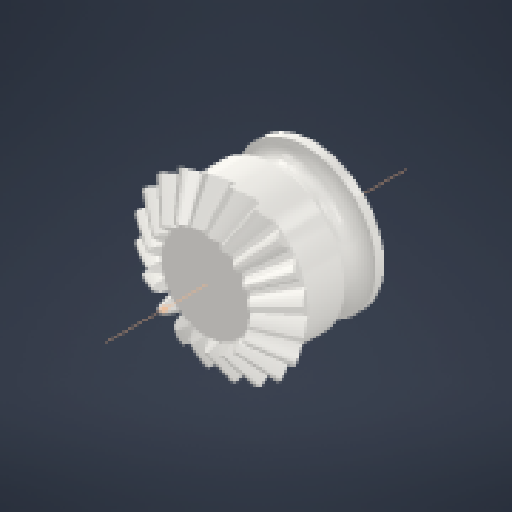
# Autodesk Inventor part: Bevel Gear2
Saved by Autodesk Inventor 2023.4 (Build 274418000, 418)
## iProperties
CustomPartVersion: 1
Created: 2025-10-03
Part Number: Bevel Gear2
Material: Steel, Mild
Document SubType Name: Modeling
Designer: Malthe Sennels
Categories: <?xml version="1.0" encoding="UTF-16"?> <MemberInstance><Categories><FamilyTemplate><FamilyTemplateParameter ValueType="xs:double" Id="1" ObjectReferenceKey="da_z" ObjectType="kUserParameterObject"/><FamilyTemplateParameter ValueType="xs:double" Id="2" ObjectReferenceKey="da_b" ObjectType="kUserParameterObject"/><FamilyTemplateParameter ValueType="xs:double" Id="3" ObjectReferenceKey="da_beta" ObjectType="kUserParameterObject"/><FamilyTemplateParameter ValueType="xs:double" Id="4" ObjectReferenceKey="da_dae" ObjectType="kUserParameterObject"/><FamilyTemplateParameter ValueType="xs:double" Id="5" ObjectReferenceKey="da_ve" ObjectType="kUserParameterObject"/><FamilyTemplateParameter ValueType="xs:double" Id="6" ObjectReferenceKey="da_omega" ObjectType="kUserParameterObject"/><FamilyTemplateParameter ValueType="xs:string" Id="7" ObjectReferenceKey="EAIAABAAAAAAHwAAAAAAAIAAAAAAAAAA" ObjectType="83914240" SubObjectId="SurfaceGeometry"/></FamilyTemplate><ParamToTemplateMap><ParamToTemplate CategoryParameter="//CategoryParameter[@InternalName='046C89C9-8512-4d59-83FE-43B91F4F132A']" TemplateParameter="1"/><ParamToTemplate CategoryParameter="//CategoryParameter[@InternalName='2552DF32-E462-4b46-AEBF-C6C7768E72AC']" TemplateParameter="2"/><ParamToTemplate CategoryParameter="//CategoryParameter[@InternalName='C9EE641D-15FC-4fae-A226-E94C4372FDD7']" TemplateParameter="3"/><ParamToTemplate><ParamToTemplate CategoryParameter="//CategoryParameter[@InternalName='00B6519A-459B-49c7-AD84-2E56D39A5744']" ConstantValue="-0.000000"/></ParamToTemplate><ParamToTemplate><ParamToTemplate CategoryParameter="//CategoryParameter[@InternalName='04B31F0E-C7A6-4894-AA32-9629BEFACF47']" ConstantValue="1.000000"/></ParamToTemplate><ParamToTemplate><ParamToTemplate CategoryParameter="//CategoryParameter[@InternalName='43CBEC2E-7847-49e7-A936-2F7889FCB2D9']" ConstantValue="0.200000"/></ParamToTemplate><ParamToTemplate><ParamToTemplate CategoryParameter="//CategoryParameter[@InternalName='B1EFC894-105D-4ebd-86BF-FA20ED196853']" ConstantValue="0.300000"/></ParamToTemplate><ParamToTemplate><ParamToTemplate CategoryParameter="//CategoryParameter[@InternalName='51175063-3D10-4879-93E8-6246FE8B403D']" ConstantValue="2060000000.000000"/></ParamToTemplate><ParamToTemplate><ParamToTemplate CategoryParameter="//CategoryParameter[@InternalName='A3A52E27-4454-46a9-B0BD-C932399B70AF']" ConstantValue="0.300000"/></ParamToTemplate><ParamToTemplate CategoryParameter="//CategoryParameter[@InternalName='2A200944-5A8C-41ca-B96E-8520D2E510F1']" TemplateParameter="4"/><ParamToTemplate><ParamToTemplate CategoryParameter="//CategoryParameter[@InternalName='1A637F62-92C8-44bc-B81F-10802510B579']" ConstantValue="1.526400"/></ParamToTemplate><ParamToTemplate CategoryParameter="//CategoryParameter[@InternalName='B52DD4BE-6863-48fb-BF58-89EF6F9EC65C']" TemplateParameter="5"/><ParamToTemplate><ParamToTemplate CategoryParameter="//CategoryParameter[@InternalName='3956BFF2-84D2-457d-93C2-9B0613DEBA67']" ConstantValue="0.482400"/></ParamToTemplate><ParamToTemplate CategoryParameter="//CategoryParameter[@InternalName='739CFA02-461B-4bf8-8049-181FCAD8B28F']" TemplateParameter="6"/><ParamToTemplate><ParamToTemplate CategoryParameter="//CategoryParameter[@InternalName='A27E999F-E2CE-4481-8A2A-EBF499C4C3C5']" ConstantValue="-0.000000"/></ParamToTemplate><ParamToTemplate><ParamToTemplate CategoryParameter="//CategoryParameter[@InternalName='9E1B4470-B2D3-4ff1-B813-535BB4CDF51A']" ConstantValue="3520000.000000"/></ParamToTemplate><ParamToTemplate><ParamToTemplate CategoryParameter="//CategoryParameter[@InternalName='F8452263-BFF6-458c-9FB1-07C4B99E95CD']" ConstantValue="11400000.000000"/></ParamToTemplate><ParamToTemplate><ParamToTemplate CategoryParameter="//CategoryParameter[@InternalName='3E3BB259-FD49-497f-8171-6EBC954A3479']" ConstantValue="2.000000"/></ParamToTemplate><ParamToTemplate CategoryParameter="//CategoryParameter[@InternalName='27C3BAF2-7550-4e4b-AE2C-0DB134B7D9B7']" TemplateParameter="7"/></ParamToTemplateMap><Category DisplayName="Gear" InternalName="DC85795E-93AB-48d5-8EEE-5A27447B64BD" Mnemonic="Gear"><CategoryParameter DisplayName="z" InternalName="046C89C9-8512-4d59-83FE-43B91F4F132A" Mnemonic="z"/><CategoryParameter DisplayName="b" InternalName="2552DF32-E462-4b46-AEBF-C6C7768E72AC" Mnemonic="b"/><CategoryParameter DisplayName="||b|" InternalName="C9EE641D-15FC-4fae-A226-E94C4372FDD7" Mnemonic="beta"/><CategoryParameter DisplayName="x" InternalName="00B6519A-459B-49c7-AD84-2E56D39A5744" Mnemonic="x"/><CategoryParameter DisplayName="a*" InternalName="04B31F0E-C7A6-4894-AA32-9629BEFACF47" Mnemonic="a"/><CategoryParameter DisplayName="c*" InternalName="43CBEC2E-7847-49e7-A936-2F7889FCB2D9" Mnemonic="c"/><CategoryParameter DisplayName="r|.f|*" InternalName="B1EFC894-105D-4ebd-86BF-FA20ED196853" Mnemonic="rf"/><CategoryParameter DisplayName="E" InternalName="51175063-3D10-4879-93E8-6246FE8B403D" Mnemonic="E"/><CategoryParameter DisplayName="||m|" InternalName="A3A52E27-4454-46a9-B0BD-C932399B70AF" Mnemonic="mi"/><Category DisplayName="BevelGear" InternalName="0C98F69A-0C2B-4791-B2FE-7691BB227E77" Mnemonic="BevelGear"><CategoryParameter DisplayName="d|.ae|" InternalName="2A200944-5A8C-41ca-B96E-8520D2E510F1" Mnemonic="dae"/><CategoryParameter DisplayName="d|.ai|" InternalName="1A637F62-92C8-44bc-B81F-10802510B579" Mnemonic="dai"/><CategoryParameter DisplayName="A|.e|" InternalName="B52DD4BE-6863-48fb-BF58-89EF6F9EC65C" Mnemonic="ve"/><CategoryParameter DisplayName="A|.i|" InternalName="3956BFF2-84D2-457d-93C2-9B0613DEBA67" Mnemonic="vi"/><CategoryParameter DisplayName="||S|" InternalName="739CFA02-461B-4bf8-8049-181FCAD8B28F" Mnemonic="omega"/><CategoryParameter DisplayName="x|.t|" InternalName="A27E999F-E2CE-4481-8A2A-EBF499C4C3C5" Mnemonic="xt"/><CategoryParameter DisplayName="||s||.Flim|" InternalName="9E1B4470-B2D3-4ff1-B813-535BB4CDF51A" Mnemonic="sFlim"/><CategoryParameter DisplayName="||s||.Hlim|" InternalName="F8452263-BFF6-458c-9FB1-07C4B99E95CD" Mnemonic="sHlim"/><CategoryParameter DisplayName="type" InternalName="3E3BB259-FD49-497f-8171-6EBC954A3479" Mnemonic="type"/><CategoryParameter DisplayName="PitchDiameter" InternalName="27C3BAF2-7550-4e4b-AE2C-0DB134B7D9B7" Mnemonic="IDS_PITCHDIAM"/></Category></Category></Categories></MemberInstance>
Mass: 60.9118 g
Surface Area: 34.3074 cm^2
Volume: 7.7496 cm^3
Density: 7.86 g/cm^3
Appearance: Steel
Author: Malthe Sennels
Autodesk Inventor part; units mm, degrees
ref_plane "Mesh Plane2" through (0, 0, 0) normal (0.9876883, 0.1564345, 0) x (0, 0, 1)
sketch "Teeth Body Sketch" plane through (0, 0, 0) normal (1, 0, 0) x (0, 1, 0)
  line L0 (0, 0) -> (11.136, -10.152) construction
  line L1 (11.136, -10.152) -> (12.72, -8.04)
  line L2 (12.72, -8.04) -> (0, 0) construction
  line L3 (12, -9) -> (0, 0) construction
  line L4 (6.6816, -6.0912) -> (7.632, -4.824)
  line L5 (11.136, -10.152) -> (6.6816, -6.0912)
  line L6 (12.72, -8.04) -> (7.632, -4.824)
  line L7 (0, -39.386751) -> (0, 6.564458)
  line L8 (0, -9) -> (12.72, -9) construction
  dimension "d0" = 24
  dimension "d1" = 22.272
  dimension "d2" = 25.44
  dimension "d3" = 6
  dimension "d4" = 8.04
  constraints: 16 end point, 4 point on line, 3 perpendicular, 2 collinear, 1 horizontal alignment, 1 vertical alignment
  measures "d0" diameter of L3.start L7
  measures "d1" diameter of L0.end L7
  measures "d2" diameter of L1.end L7
  measures "d3" distance between parallel lines of L1 L4
  measures "d4" vertical distance of L1.end L0.start
revolve "Teeth Body" add sketch "Teeth Body Sketch" angle 360 about axis through (0, 0, 0) along (0, 0, 1)
ref_plane "Tooth Plane" through (0, 12, -9) normal (0, -0.8, 0.6) x (1, 0, 0)
sketch "Start Sketch" plane through (0, 12, -9) normal (0, -0.8, 0.6) x (1, 0, 0)
  line L0 (0, -23.505131) -> (0, 10.644758)
  arc A0 (-0.371395, -1.7568) -> (-2.200263, 1.881657) centre (-8.21899, -3.422521) ccw
  arc A1 (2.200263, 1.881657) -> (0.371395, -1.7568) centre (8.21899, -3.422521) ccw
  line L1 (-0.371395, -1.7568) -> (0.371395, -1.7568)
  arc A2 (2.200263, 1.881657) -> (-2.200263, 1.881657) centre (0, -20) ccw
  dimension "d7" = 8.02243
  dimension "d8" = 8.21899
  dimension "d9" = 16.57748
  dimension "d57" = 21.992
  dimension "d58" = 18.2432
  constraints: 6 point on circle, 3 centre point, 3 symmetric about line, 2 end point, 1 coincident, 1 perpendicular, 1 other
  measures "d7" radius of A0
  measures "d8" horizontal distance of point (0, -20) A0.centre
  measures "d9" vertical distance of point (0, -20) A0.centre
  measures "d57" radius of A2
  measures "d58" distance from line of A2.centre L1
sketch "End Sketch" plane through (0, 7.0944, -5.3208) normal (0, -0.8, 0.6) x (1, 0, 0)
  line L0 (0, -15.35404) -> (0, 6.953444)
  arc A0 (-0.219569, -1.03862) -> (-1.300796, 1.112436) centre (-4.859067, -2.023395) ccw
  arc A1 (1.300796, 1.112436) -> (0.219569, -1.03862) centre (4.859067, -2.023395) ccw
  line L1 (-0.219569, -1.03862) -> (0.219569, -1.03862)
  arc A2 (1.300796, 1.112436) -> (-1.300796, 1.112436) centre (0, -11.824) ccw
  dimension "d12" = 4.74286
  dimension "d15" = 4.85907
  dimension "d16" = 9.80061
  dimension "d59" = 13.00167
  dimension "d60" = 10.78538
  constraints: 6 point on circle, 3 centre point, 3 symmetric about line, 2 end point, 1 coincident, 1 other
  measures "d12" radius of A0
  measures "d15" horizontal distance of A0.centre point (0, -11.824)
  measures "d16" vertical distance of A0.centre point (0, -11.824)
  measures "d59" radius of A2
  measures "d60" distance from line of A2.centre L1
loft "Loft" cut profiles "Start Sketch", "End Sketch"
pattern_circular "Circular Pattern" count 20 over 360 about axis through (0, 0, 0) along (0, 0, 1) of "Loft"
ref_plane "End Plane" through (0, 7.0944, -5.3208) normal (0, -0.8, 0.6) x (1, 0, 0)
sketch3d "3D Sketch Right"
ref_plane "End Plane Right" through (-1.634531, 6.903537, -5.3208) normal (0.1843179, -0.7784773, 0.6) x (0.9730966, 0.2303973, 0)
sketch "End Sketch Right" plane through (-1.634531, 6.903537, -5.3208) normal (0.1843179, -0.7784773, 0.6) x (0.9730966, 0.2303973, 0)
  arc A0 (-0.219569, -1.03862) -> (-1.300796, 1.112436) centre (-4.859067, -2.023395) ccw
  line L0 (0, -17.83564) -> (0, 9.435033)
  arc A1 (1.300796, 1.112436) -> (0.219569, -1.03862) centre (4.859067, -2.023395) ccw
  line L1 (-0.219569, -1.03862) -> (0.219569, -1.03862)
  arc A2 (1.300796, 1.112436) -> (-1.300796, 1.112436) centre (0, -11.824) ccw
  dimension "d70" = 4.85907
  dimension "d71" = 9.80061
  dimension "d72" = 4.74286
  dimension "d73" = 10.78538
  dimension "d74" = 13.00167
  constraints: 6 point on circle, 3 centre point, 3 symmetric about line, 2 end point, 1 coincident, 1 perpendicular, 1 other
  measures "d70" horizontal distance of A2.centre A0.centre
  measures "d71" vertical distance of point (0, -11.824) A0.centre
  measures "d72" radius of A0
  measures "d73" distance from line of point (0, -11.824) L1
  measures "d74" radius of A2
feature "Loft Right" [suppressed]
pattern_circular "Circular Pattern Right" [suppressed]
sketch3d "3D Sketch Left"
ref_plane "End Plane Left" through (1.65692, 6.903537, -5.330829) normal (-0.1866285, -0.7775854, 0.6004421) x (0.972385, -0.2333825, 0)
sketch "End Sketch Left" plane through (1.65692, 6.903537, -5.330829) normal (-0.1866285, -0.7775854, 0.6004421) x (0.972385, -0.2333825, 0)
  line L0 (0, -30.720669) -> (0, 13.697946)
  arc A0 (-0.219569, -1.033716) -> (-1.300796, 1.117339) centre (-4.859067, -2.018491) ccw
  arc A1 (1.300796, 1.117339) -> (0.219569, -1.033716) centre (4.859067, -2.018491) ccw
  line L1 (-0.219569, -1.033716) -> (0.219569, -1.033716)
  ellipse E0 centre (0, -3.857599) end of major axis (7.632, -3.857599) minor radius 4.582574
  arc A2 (1.300796, 1.117339) -> (-1.300796, 1.117339) centre (0, -11.819096) ccw
  dimension "d56" = 4.58257
  dimension "d30" = 4.74286
  dimension "d31" = 4.85907
  dimension "d32" = 9.80061
  dimension "d61" = 13.00167
  dimension "d62" = 10.78538
  constraints: 6 point on circle, 3 centre point, 3 symmetric about line, 2 end point, 1 coincident, 2 other
  measures "d30" radius of A0
  measures "d31" horizontal distance of point (0, -11.819) A0.centre
  measures "d32" vertical distance of A0.centre point (0, -11.819)
  measures "d61" radius of A2
  measures "d62" distance from line of point (0, -11.819) L1
feature "Loft Left" [suppressed]
pattern_circular "Circular Pattern Left" [suppressed]
sketch "Body Sketch" plane through (0, 0, 0) normal (1, 0, 0) x (0, 1, 0)
  line L0 (0, -35.037536) -> (0, -19.530831)
  line L1 (11.136, -10.152) -> (6.6816, -6.0912)
  line L2 (6.6816, -6.0912) -> (0, -6.0912)
  line L3 (11.136, -10.152) -> (0, -10.152)
  constraints: 4 end point, 2 perpendicular, 2 point on line
sketch "Body Sketch outline for Fix Body" plane through (0, 0, 0) normal (1, 0, 0) x (0, 1, 0)
  line L0 (0, -10.152) -> (11.136, -10.152)
  line L1 (0, -6.0912) -> (0, -10.152)
  line L2 (6.6816, -6.0912) -> (0, -6.0912)
  line L3 (11.136, -10.152) -> (6.6816, -6.0912)
revolve "Fix Body" add sketch "Body Sketch outline for Fix Body" angle 360 about axis through (0, 0, 0) along (0, 0, 1)
sketch "Sketch6" plane through (0, 0, 0) normal (1, 0, 0) x (0, 1, 0)
  line L0 (12, -9) -> (0, 0)
  line L1 (0, -37.799919) -> (0, 6.299986)
surface revolve "Pitch Diameter" sketch "Sketch6" angle 360 about axis through (0, 0, 0) along (0, 0, 1) shown no curves L0
sketch "Sketch8" plane through (0, 0, 0) normal (0, 1, 0) x (-1, 0, 0)
  line L0 (0.443648, -10.152) -> (-0.443648, -10.152)
  line L1 (-0.443648, -10.152) -> (-3.016547, -10.152)
  line L2 (-3.016547, -10.152) -> (-3.860416, -10.152)
  line L3 (-3.860416, -10.152) -> (-6.181461, -10.152)
  line L4 (-6.181461, -10.152) -> (-6.899299, -10.152)
  line L5 (-6.899299, -10.152) -> (-8.741291, -10.152)
  line L6 (-8.741291, -10.152) -> (-9.262831, -10.152)
  line L7 (-9.262831, -10.152) -> (-10.445462, -10.152)
  line L8 (-10.445462, -10.152) -> (-10.719652, -10.152)
  line L9 (-10.719652, -10.152) -> (-11.127159, -10.152)
  line L10 (-11.127159, -10.152) -> (-11.127159, -10.152)
  line L11 (-11.127159, -10.152) -> (-10.719652, -10.152)
  line L12 (-10.719652, -10.152) -> (-10.445462, -10.152)
  line L13 (-10.445462, -10.152) -> (-9.262831, -10.152)
  line L14 (-9.262831, -10.152) -> (-8.741291, -10.152)
  line L15 (-8.741291, -10.152) -> (-6.899299, -10.152)
  line L16 (-6.899299, -10.152) -> (-6.181461, -10.152)
  line L17 (-6.181461, -10.152) -> (-3.860416, -10.152)
  line L18 (-3.860416, -10.152) -> (-3.016547, -10.152)
  line L19 (-3.016547, -10.152) -> (-0.443648, -10.152)
  line L20 (-0.443648, -10.152) -> (0.443648, -10.152)
  line L21 (0.443648, -10.152) -> (3.016547, -10.152)
  line L22 (3.016547, -10.152) -> (3.860416, -10.152)
  line L23 (3.860416, -10.152) -> (6.181461, -10.152)
  line L24 (6.181461, -10.152) -> (6.899299, -10.152)
  line L25 (6.899299, -10.152) -> (8.741291, -10.152)
  line L26 (8.741291, -10.152) -> (9.262831, -10.152)
  line L27 (9.262831, -10.152) -> (10.445462, -10.152)
  line L28 (10.445462, -10.152) -> (10.719652, -10.152)
  line L29 (10.719652, -10.152) -> (11.127159, -10.152)
  line L30 (11.127159, -10.152) -> (11.127159, -10.152)
  line L31 (11.127159, -10.152) -> (10.719652, -10.152)
  line L32 (10.719652, -10.152) -> (10.445462, -10.152)
  line L33 (10.445462, -10.152) -> (9.262831, -10.152)
  line L34 (9.262831, -10.152) -> (8.741291, -10.152)
  line L35 (8.741291, -10.152) -> (6.899299, -10.152)
  line L36 (6.899299, -10.152) -> (6.181461, -10.152)
  line L37 (6.181461, -10.152) -> (3.860416, -10.152)
  line L38 (3.860416, -10.152) -> (3.016547, -10.152)
  line L39 (3.016547, -10.152) -> (0.443648, -10.152)
  line L40 (-11.127159, -10.152) -> (0, -10.152)
  line L41 (0, -10.152) -> (0, -16.152)
  line L42 (0, -16.152) -> (-10.6, -16.152) construction
  arc A0 (-10.6, -32.951902) -> (-10.6, -28.319139) centre (-10.8, -30.63552) ccw
  arc A1 (-10.6, -20.802) -> (-10.6, -16.152) centre (-10.6, -18.477) ccw
  line L43 (-10.6, -18.477) -> (-10.6, -20.802) construction
  line L44 (-10.6, -18.477) -> (-10.6, -16.152) construction
  line L45 (-10.6, -20.802) -> (0, -20.802) construction
  line L46 (0, -20.802) -> (0, -22.082)
  line L47 (0, -22.082) -> (-10.6, -22.082)
  line L48 (-10.6, -22.082) -> (-10.6, -20.802)
  line L49 (-10.6, -34.13552) -> (-10.6, -32.951902)
  line L50 (0, -20.802) -> (0, -16.152)
  line L51 (-0.443648, -10.152) -> (0.443648, -10.152)
  line L52 (-10.6, -16.152) -> (-10.6, -10.152)
  point P0 (0, 0)
  point P1 (-10.923406, -10.152)
  point P2 (0, -10.152)
  point P3 (0, -10.152)
  dimension "d94" = 180
  dimension "d95" = 2.325
  dimension "d96" = 1.28
  dimension "d97" = 6
  dimension "d99" = 10.6
  constraints: 24 end point, 4 point on circle, 3 parallel, 3 perpendicular, 2 centre point, 2 horizontal, 2 midpoint, 2 point on line, 2 vertical, 1 collinear, 5 other
  measures "d94" angle of L44 L43
  measures "d95" radius of A1
  measures "d96" distance of L47.end L43.end
  measures "d97" distance from line of point (-10.923, -10.152) L42
  measures "d99" distance of L46.end L47.end
revolve "Revolution3" add sketch "Sketch8" angle 360 about axis through (0, 0, -10.152) along (0, 0, -1)
sketch "Sketch9" plane through (0, 0, -22.082) normal (0, 0, -1) x (-1, 0, 0)
  line L0 (0, 0) -> (0, -4.5) construction
  circle A0 centre (0, -4.5) radius 2.2
  circle A1 centre (0, 4.5) radius 2.2
  dimension "d100" = 4.5
  dimension "d101" = 4.4
  dimension "d104" = 360
  constraints: 2 centre point, 2 end point, 1 coincident, 1 vertical, 5 other
  measures "d100" distance of L0.start L0.end
  measures "d101" diameter of A0
extrude "Extrusion1" cut sketch "Sketch9" against normal blind 10
equation "\"d0\" = da_de"
equation "\"d1\" = da_dfe"
equation "\"d2\" = da_dae"
equation "\"d3\" = da_b"
equation "\"d4\" = da_ve"
equation "\"d7\" = fd_rr"
equation "\"d8\" = fd_x"
equation "\"d9\" = fd_y"
equation "\"d57\" = 0.5 * fd_dva + 0.3 * da_he"
equation "\"d58\" = 0.5 * fd_dva - 1.12 * da_he"
equation "\"da_teethtype\" = 0"
equation "\"da_b\" = 6"
equation "\"da_de\" = 24"
equation "\"da_dae\" = 25.44"
equation "\"da_dfe\" = 22.272"
equation "\"da_le\" = 15"
equation "\"da_omega\" = 90deg"
equation "\"da_beta\" = 0"
equation "\"da_delta\" = 53.130102deg"
equation "\"da_alpha\" = 22.5deg"
equation "\"da_he\" = 2.64"
equation "\"da_ve\" = 8.04"
equation "\"da_zv\" = 33.333333"
equation "\"fd_loft\" = da_b + 0.05 * da_he"
equation "\"fd_x\" = fd_x1 + fd_x2"
equation "\"fd_y\" = fd_y1 - fd_y2"
equation "\"fd_dd\" = fd_dva - 0.8 * da_he"
equation "\"d11\" = fd_loft"
equation "\"da_dm\" = 19.2"
equation "\"da_x\" = 0"
equation "\"da_m\" = 1.2"
equation "\"d50\" = da_omega"
equation "\"fd_rr\" = 8.02243"
equation "\"fd_dva\" = 42.4"
equation "\"fd_x1\" = 0.952589"
equation "\"fd_x2\" = 7.266401"
equation "\"fd_y1\" = 19.977301"
equation "\"fd_y2\" = 3.399823"
body "Solid1"
body "Srf1"
